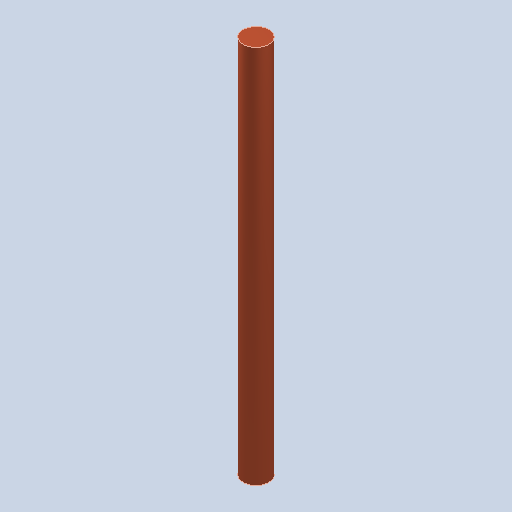
# Autodesk Inventor part: pret22mm
Saved by Autodesk Inventor 2024.2 (Build 282272000, 272)
## iProperties
Created: 2024-01-20
Part Number: pret22mm
Material: Miedź
Document SubType Name: Modeling
Designer: Konrad
Density: 8.94 g/cm^3
Appearance: Miedź — satynowa
Author: Konrad
Autodesk Inventor part; units mm, degrees
ref_plane "YZ Plane" through (0, 0, 0) normal (1, 0, 0) x (0, 1, 0)
ref_plane "XZ Plane" through (0, 0, 0) normal (0, 1, 0) x (-1, 0, 0)
ref_plane "XY Plane" through (0, 0, 0) normal (0, 0, 1) x (1, 0, 0)
sketch "Szkic1" plane through (0, 0, 0) normal (0, 1, 0) x (-1, 0, 0)
  circle A0 centre (0, 0) radius 0.75
  dimension "d0" = 1.5
  constraints: 1 centre point, 1 coincident
  measures "d0" diameter of A0
extrude "Wyciągnięcie proste1" add sketch "Szkic1" along normal blind 22
